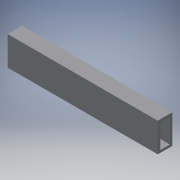
# Autodesk Inventor part: snoRail
Saved by Autodesk Inventor 2016 (Build 200138000, 138)
## iProperties
Created: 2016-01-28
Part Number: snoRail
Material: Generic
Document SubType Name: Modeling
Designer: bbier
Density: 1 g/cm^3
Appearance: Default
Author: bbier
Autodesk Inventor part; units mm, degrees
ref_plane "YZ Plane" through (0, 0, 0) normal (1, 0, 0) x (0, 1, 0)
ref_plane "XZ Plane" through (0, 0, 0) normal (0, 1, 0) x (-1, 0, 0)
ref_plane "XY Plane" through (0, 0, 0) normal (0, 0, 1) x (1, 0, 0)
sketch "Sketch1" plane through (0, 0, 0) normal (1, 0, 0) x (0, 1, 0)
  line L0 (34.925, -3.175) -> (3.175, -3.175)
  line L1 (3.175, -3.175) -> (3.175, -15.875)
  line L2 (3.175, -15.875) -> (34.925, -15.875)
  line L3 (34.925, -15.875) -> (34.925, -3.175)
  line L4 (0, 0) -> (38.1, 0)
  line L5 (38.1, 0) -> (38.1, -19.05)
  line L6 (38.1, -19.05) -> (0, -19.05)
  line L7 (0, -19.05) -> (0, 0)
  dimension "d6" = 38.1
  dimension "d7" = 19.05
  constraints: 16 end point, 4 parallel, 2 horizontal, 2 perpendicular
  measures "d6" distance of L5.end L6.end
  measures "d7" distance of L4.end L5.end
extrude "Extrusion1" add sketch "Sketch1" along normal blind 25.4
thicken "Thicken1" operation add thickness 190.5 both sides no extend neighbours yes toward (1, 0, 0) faces at (25.4, 13.7583, -17.9917)
thicken "Thicken2" operation add thickness 19.05 both sides no extend neighbours yes toward (-1, 0, 0) faces at (215.9, 13.7583, -17.9917)
body "Solid1"
